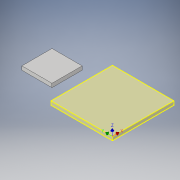
# Autodesk Inventor part: Calibration Inch Square
Saved by Autodesk Inventor 2018 (Build 220112000, 112)
## iProperties
Created: 2017-09-27
Part Number: Calibration Inch Square
Material: Generic
Document SubType Name: Modeling
Designer: Samuel Clay
Density: 1 g/cm^3
Appearance: Default
Author: Samuel Clay
Autodesk Inventor part; units mm, degrees
ref_plane "YZ Plane" through (0, 0, 0) normal (1, 0, 0) x (0, 1, 0)
ref_plane "XZ Plane" through (0, 0, 0) normal (0, 1, 0) x (-1, 0, 0)
ref_plane "XY Plane" through (0, 0, 0) normal (0, 0, 1) x (1, 0, 0)
sketch "Sketch1" plane through (0, 0, 0) normal (0, 1, 0) x (-1, 0, 0)
  line L0 (12.7, -12.7) -> (-12.7, -12.7)
  line L1 (-12.7, -12.7) -> (-12.7, 12.7)
  line L2 (-12.7, 12.7) -> (12.7, 12.7)
  line L3 (12.7, 12.7) -> (12.7, -12.7)
  line L4 (12.7, -12.7) -> (-12.7, 12.7) construction
  line L5 (-12.7, -12.7) -> (12.7, 12.7) construction
  point P0 (0, 0)
  dimension "d0" = 25.4
  dimension "d1" = 25.4
  constraints: 12 end point, 2 midpoint, 2 parallel, 1 horizontal, 1 perpendicular
  measures "d0" distance of L1.end L2.end
  measures "d1" distance of L0.end L1.end
extrude "Extrusion1" add sketch "Sketch1" along normal blind 3.175
sketch "Sketch2" plane through (0, 0, 0) normal (0, 1, 0) x (-1, 0, 0)
  line L0 (-24.8666, -25.9334) -> (-76.7334, -25.9334)
  line L1 (-76.7334, -25.9334) -> (-76.7334, 25.9334)
  line L2 (-76.7334, 25.9334) -> (-24.8666, 25.9334)
  line L3 (-24.8666, 25.9334) -> (-24.8666, -25.9334)
  line L4 (-24.8666, -25.9334) -> (-76.7334, 25.9334) construction
  line L5 (-76.7334, -25.9334) -> (-24.8666, 25.9334) construction
  point P0 (0, 0)
  point P1 (-50.8, 0)
  point P2 (-50.8, 0)
  dimension "d4" = 51.8668
  dimension "d5" = 51.8668
  dimension "d6" = 50.8
  constraints: 12 end point, 3 midpoint, 2 parallel, 1 horizontal, 1 horizontal alignment, 1 perpendicular
  measures "d4" distance of L1.end L2.end
  measures "d5" distance of L0.end L1.end
  measures "d6" distance of point (0, 0) point (-50.8, 0)
extrude "Extrusion2" add sketch "Sketch2" along normal blind 3.175 separate body
body "Solid1"
body "Solid2"
